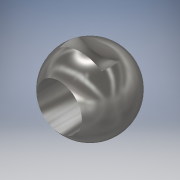
# Autodesk Inventor part: Ball
Saved by Autodesk Inventor 2018 (Build 220112000, 112)
## iProperties
Created: 2017-09-12
Part Number: Ball
Material: Stainless Steel
Document SubType Name: Modeling
Designer: kurtis
Density: 8 g/cm^3
Appearance: Semi-Polished
Author: kurtis
Autodesk Inventor part; units mm, degrees
ref_plane "YZ Plane" through (0, 0, 0) normal (1, 0, 0) x (0, 1, 0)
ref_plane "XZ Plane" through (0, 0, 0) normal (0, 1, 0) x (-1, 0, 0)
sketch "Sketch1" plane through (0, 0, 0) normal (0, 0, 1) x (1, 0, 0)
  line L0 (-16, -27) -> (-16, 27)
  line L1 (-16, 27) -> (16, 27)
  line L2 (16, 27) -> (16, -27)
  line L3 (16, -27) -> (-16, -27)
  line L4 (-16, -27) -> (16, 27) construction
  line L5 (-16, 27) -> (16, -27) construction
  line L6 (0, 27) -> (0, -27) construction
  arc A0 (-16, 21.7486) -> (-16, -21.7486) centre (0, 0) ccw
  arc A1 (16, -21.7486) -> (16, 21.7486) centre (0, 0) ccw
  line L7 (0, 0) -> (51.7536, 0) construction
  dimension "d1" = 32
  dimension "d2" = 27
  constraints: 16 end point, 4 midpoint, 4 point on circle, 4 point on line, 2 centre point, 2 parallel, 2 tangent, 1 coincident, 1 horizontal, 1 perpendicular, 1 vertical
  measures "d1" distance of L0.end L1.end
  measures "d2" radius of A1
revolve "Revolution1" add sketch "Sketch1" angle 360 about axis through (0, 27, 0) along (0, -1, 0) contours A0 L0
ref_plane "Work Plane5" through (16, -27, 0) normal (0, -1, 0) x (1, 0, 0)
ref_plane "Work Plane7" through (0, 0, 0) normal (0, -1, 0) x (1, 0, 0)
ref_plane "Work Plane6" through (0, 27, 0) normal (0, -1, 0) x (1, 0, 0)
sketch "Sketch4" plane through (0, 0, 0) normal (0, -1, 0) x (1, 0, 0)
  line L0 (0, 0) -> (0, 50) construction
  arc A0 (-15.582, 22.05) -> (15.582, 22.05) centre (0, 50) ccw
  circle A1 centre (0, 0) radius 27
  line L1 (0, 50) -> (-15.582, 22.05) construction
  line L2 (0, 50) -> (15.582, 22.05) construction
  dimension "d10" = 50
  dimension "d11" = 32
  dimension "d12" = 58.279
  dimension "d13" = 24.3468
  dimension "d14" = 0
  constraints: 6 end point, 4 point on circle, 2 centre point, 2 coincident, 1 vertical
  measures "d10" distance of L0.start L0.end
  measures "d11" radius of A0
  measures "d12" angle of L2 L1
  measures "d13" distance from line of point (0, 0) L2
  measures "d14" distance from line of point (0, 0) L0
extrude "Extrusion1" cut sketch "Sketch4" along normal mid plane 13 contours A1 A0 picked at (1.0831, 23.9191)
body "Solid1"
